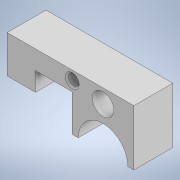
# Autodesk Inventor part: Pieza modelo
Saved by Autodesk Inventor 2022 (Build 260153000, 153)
## iProperties
Created: 2022-07-28
Part Number: Pieza modelo
Material: Generic
Document SubType Name: Modeling
Designer: iemcc
Density: 1 g/cm^3
Appearance: Default
Author: iemcc
Autodesk Inventor part; units mm, degrees
ref_plane "YZ Plane" through (0, 0, 0) normal (1, 0, 0) x (0, 1, 0)
ref_plane "XZ Plane" through (0, 0, 0) normal (0, 1, 0) x (-1, 0, 0)
ref_plane "XY Plane" through (0, 0, 0) normal (0, 0, 1) x (1, 0, 0)
sketch "Sketch1" plane through (0, 0, 0) normal (0, 0, 1) x (1, 0, 0)
  line L0 (-16.6163, 0) -> (-16.6163, -6.1597)
  line L1 (-16.6163, -6.1597) -> (-11.989, -6.1597)
  line L2 (-11.989, -6.1597) -> (-11.989, -3.0799)
  line L3 (-11.989, -3.0799) -> (-5.9795, -3.0799)
  line L4 (-5.9795, -3.0799) -> (-5.9795, -9.1044)
  line L5 (4.1165, -9.1044) -> (4.1165, 0)
  line L6 (4.1165, 0) -> (-16.6163, 0)
  arc A0 (3.1288, -9.1044) -> (-4.9917, -9.1044) centre (-0.9315, -9.1044) ccw
  line L7 (-5.9795, -9.1044) -> (-4.9917, -9.1044)
  line L8 (3.1288, -9.1044) -> (4.1165, -9.1044)
  circle A1 centre (-0.9315, -2.2963) radius 1.7633
  point P0 (0, 0)
  point P1 (-16.6163, -3.0799)
  constraints: 18 end point, 9 perpendicular, 2 centre point, 2 point on circle, 1 midpoint, 1 point on line, 1 vertical
extrude "Extrusion1" add sketch "Sketch1" along normal mid plane 6.3627
sketch "Sketch3" plane through (0, 0, 3.1814) normal (0, 0, 1) x (1, 0, 0)
  point P0 (0, 0)
  point P1 (-5.9778, -1.4956)
hole "Hole1" at (-5.9778, -1.4956, 3.1814) direction (0, 0, -1) diameter 1.778 end through all countersink diameter 2.286 countersink angle 82
body "Solid1"
